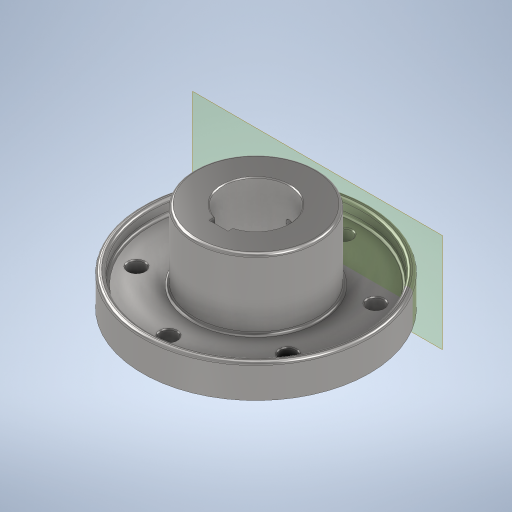
# Autodesk Inventor part: S2spojkav3
Saved by Autodesk Inventor 2023 (Build 270158000, 158)
## iProperties
Created: 2023-05-05
Part Number: S2spojkav3
Material: 42 2420
Document SubType Name: Modeling
Designer: S21Suk
Density: 7.85 g/cm^3
Appearance: Semi-Polished
Description: Kotoučová spojka
Mass: 12576.1 g
Surface Area: 1712.28 cm^2
Volume: 1602.05 cm^3
Material: ČSN 42 2420
Appearance: Pololeštěná
Mass: 12572.3 g
Surface Area: 1713.08 cm^2
Volume: 1601.57 cm^3
Polotovar: Odlitek
Author: S21Suk
Autodesk Inventor part; units mm, degrees
ref_plane "YZ Plane" through (0, 0, 0) normal (1, 0, 0) x (0, 1, 0)
ref_plane "XZ Plane" through (0, 0, 0) normal (0, 1, 0) x (-1, 0, 0)
ref_plane "XY Plane" through (0, 0, 0) normal (0, 0, 1) x (1, 0, 0)
sketch "Náčrt1" plane through (0, 0, 0) normal (0, 1, 0) x (-1, 0, 0)
  circle A0 centre (0, 0) radius 120
  circle A1 centre (0, 0) radius 112.5
  circle A2 centre (0, 0) radius 35
  circle A3 centre (0, 0) radius 65
  circle A4 centre (0, -92.5) radius 8.5
  line L0 (0, -65) -> (0, -92.5) construction
  circle A5 centre (80.1073, -46.25) radius 8.5
  circle A6 centre (80.1073, 46.25) radius 8.5
  circle A7 centre (0, 92.5) radius 8.5
  circle A8 centre (-80.1073, 46.25) radius 8.5
  circle A9 centre (-80.1073, -46.25) radius 8.5
  dimension "d3" = 130
  dimension "d0" = 240
  dimension "d1" = 225
  dimension "d2" = 70
  dimension "d59" = 17
  dimension "d61" = 27.5
  dimension "d64" = 360
  dimension "d67" = 185
  constraints: 9 centre point, 4 coincident, 2 end point, 1 vertical, 1 vertical alignment, 15 other
  measures "d0" diameter of A0
  measures "d1" diameter of A1
  measures "d2" diameter of A2
  measures "d59" diameter of A4
  measures "d61" distance of L0.start L0.end
  measures "d67" distance of L0.end A7.centre
extrude "Vysunutí1" add sketch "Náčrt1" along normal blind 95 contours A3
extrude "Vysunutí2" add sketch "Náčrt1" along normal blind 21 contours A1
extrude "Vysunutí3" add sketch "Náčrt1" along normal blind 35 contours A0
sketch "Náčrt3" plane through (0, 0, 0) normal (0, -1, 0) x (1, 0, 0)
  circle A0 centre (0, 0) radius 35 projected
  line L0 (10, 39.6) -> (-10, 39.6)
  line L1 (-10, 39.6) -> (-10, 27.6)
  line L2 (-10, 27.6) -> (10, 27.6)
  line L3 (10, 27.6) -> (10, 39.6)
  point P0 (0, 35)
  point P1 (0, 39.6)
  point P2 (0, 27.6)
  point P3 (10, 33.541)
  point P4 (-10, 33.541)
  dimension "d99" = 20
  dimension "d100" = 12
  dimension "d101" = 4.6
  dimension "d102" = 27.6
  dimension "d103" = 7.4
  constraints: 8 end point, 2 midpoint, 2 parallel, 1 horizontal, 1 perpendicular, 2 other
  measures "d99" distance of L2.end L1.end
  measures "d100" distance of L1.end L0.end
  measures "d101" distance of point (0, 39.6) point (0, 35)
  measures "d102" distance of point (0, 0) point (0, 27.6)
  measures "d103" distance of point (0, 27.6) point (0, 35)
extrude "Vysunutí5" cut sketch "Náčrt3" against normal through all contours L3 L2 L1 A0 | A0 L1 L0 L3 picked at (-1.1251, 30.0123)
fillet "Fillet1" radius 3 5 edges at (112.5, 21, 0) (65, 21, 0) (112.5, 35, 0) (120, 35, 0) (65, 95, 0)
ref_plane "Work Plane3" through (0, 0, -65) normal (0, 0, -1) x (-1, 0, 0)
chamfer "Zkosení1" distance 1 angle 45 14 edges at (0, 95, -35) (0, 0, -35) (-71.6073, 21, -46.25) (-71.6073, 21, 46.25) (88.6073, 21, 46.25) (8.5, 21, 92.5) (88.6073, 21, -46.25) (8.5, 21, -92.5) (8.5, 0, 92.5) (88.6073, 0, 46.25) (88.6073, 0, -46.25) (8.5, 0, -92.5) (-71.6073, 0, -46.25) (-71.6073, 0, 46.25)
sketch "Sketch12" plane through (0, 0, -65) normal (0, 0, -1) x (-1, 0, 0)
  circle A0 centre (0, 60) radius 4
  line L0 (120, 0) -> (-120, 0) projected
  line L1 (10, 94) -> (10, 1) projected
  point P0 (0, 0)
  dimension "d123" = 8
  dimension "d124" = 60
  dimension "d125" = 10
  constraints: 1 centre point
  measures "d123" diameter of A0
  measures "d124" distance from line of L0 A0.centre
  measures "d125" distance from line of L1 A0.centre
hole "Hole1" at (0, 60, -65) direction (0, 0, 1) diameter 6.647 depth 30 tip angle 118 thread size "M8x1.25" class "6H" standard "ISO Metric profile"
sketch "Sketch13" plane through (0, 0, 0) normal (0, -1, 0) x (1, 0, 0)
  line L0 (0, 0) -> (-125, 0)
  line L1 (-125, 0) -> (-125, -125)
  line L2 (-125, -125) -> (0, -125)
  line L3 (0, -125) -> (0, 0)
  dimension "d133" = 125
  dimension "d134" = 125
  constraints: 8 end point, 2 parallel, 1 horizontal, 1 perpendicular
  measures "d133" distance of L2.end L1.end
  measures "d134" distance of L1.end L0.end
extrude "Extrusion14" [suppressed]
